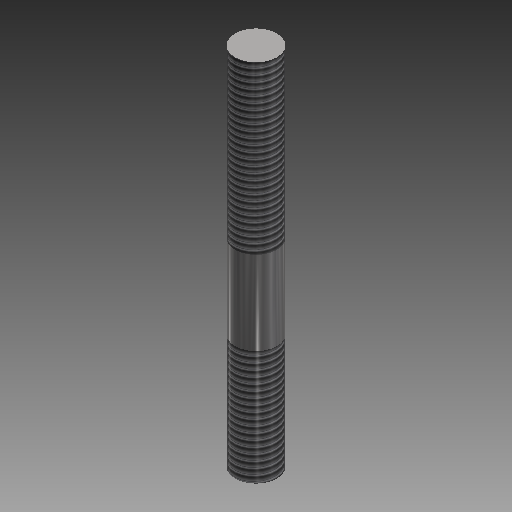
# Autodesk Inventor part: Śruba_do_widelca
Saved by Autodesk Inventor 2017 (Build 210142000, 142)
## iProperties
Created: 2016-01-12
Part Number: Śruba_do_widelca
Material: Stal nierdzewna
Document SubType Name: Modeling
Designer: graaapsik
Density: 8.08 g/cm^3
Appearance: Częściowo polerowany
Mass: 95.9518 g
Surface Area: 41.846 cm^2
Volume: 11.8752 cm^3
Author: graaapsik
Autodesk Inventor part; units mm, degrees
ref_plane "YZ Plane" through (0, 0, 0) normal (1, 0, 0) x (0, 1, 0)
ref_plane "XZ Plane" through (0, 0, 0) normal (0, 1, 0) x (-1, 0, 0)
ref_plane "XY Plane" through (0, 0, 0) normal (0, 0, 1) x (1, 0, 0)
sketch "Szkic1" plane through (0, 0, 0) normal (0, 1, 0) x (-1, 0, 0)
  circle A0 centre (0, 0) radius 6
  dimension "d0" = 12
  constraints: 1 centre point, 1 coincident
  measures "d0" diameter of A0
extrude "Wyciągnięcie proste1" add sketch "Szkic1" along normal mid plane 105
thread "Gwint1" size "M12x1.75" class "6g" standard "ANSI Metric M Profile" length 48
thread "Gwint2" size "M12x1.75" class "6g" standard "ANSI Metric M Profile" length 33
